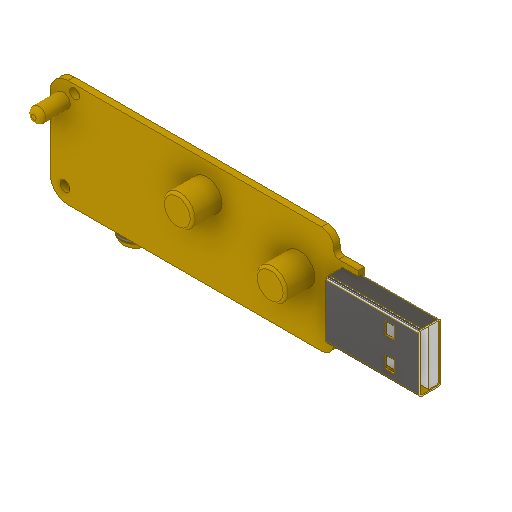
# Autodesk Inventor part: COTS_GENERIC_rtl_sdr_dongle
Saved by Autodesk Inventor 2025 (Build 290162010, 162A)
## iProperties
Created: 2018-09-08
Part Number: COTS_GENERIC_rtl_sdr_dongle
Material: Generic
Document SubType Name: Modeling
Designer: Andrzej
Density: 1 g/cm^3
Appearance: Gold
Author: Andrzej
Autodesk Inventor part; units mm, degrees
ref_plane "YZ Plane" through (0, 0, 0) normal (1, 0, 0) x (0, 1, 0)
ref_plane "XZ Plane" through (0, 0, 0) normal (0, 1, 0) x (-1, 0, 0)
ref_plane "XY Plane" through (0, 0, 0) normal (0, 0, 1) x (1, 0, 0)
sketch "Sketch1" plane through (0, 0, 0) normal (0, 0, 1) x (1, 0, 0)
  line L0 (-11.3863, 5.2126) -> (40.5137, 5.2126)
  line L1 (40.5137, -16.7874) -> (-11.3863, -16.7874)
  line L2 (-14.9863, -13.1874) -> (-14.9863, 1.6126)
  line L3 (44.0137, 1.2126) -> (48.0137, 1.2126)
  line L4 (48.0137, 1.2126) -> (48.0137, -12.7874)
  line L5 (48.0137, -12.7874) -> (44.0137, -12.7874)
  arc A0 (-14.9863, -13.1874) -> (-11.3863, -16.7874) centre (-11.3863, -13.1874) ccw
  arc A1 (-11.3863, 5.2126) -> (-14.9863, 1.6126) centre (-11.3863, 1.6126) ccw
  arc A2 (43.0137, 2.7126) -> (40.5137, 5.2126) centre (40.5137, 2.7126) ccw
  arc A3 (40.5137, -16.7874) -> (43.0137, -14.2874) centre (40.5137, -14.2874) ccw
  line L6 (43.0137, 2.7126) -> (43.0137, 2.2126)
  line L7 (43.0137, -13.7874) -> (43.0137, -14.2874)
  arc A4 (43.0137, 2.2126) -> (44.0137, 1.2126) centre (44.0137, 2.2126) ccw
  arc A5 (44.0137, -12.7874) -> (43.0137, -13.7874) centre (44.0137, -13.7874) ccw
  circle A6 centre (-11.9863, -13.7874) radius 1.05
  circle A7 centre (-9.9863, 3.6126) radius 1.05
  point P0 (0, 0)
  dimension "d3" = 14
  dimension "d4" = 4
  dimension "d7" = 3.6
  dimension "d8" = 2.5
  dimension "d9" = 1
  dimension "d10" = 2.1
  dimension "d11" = 3
  dimension "d12" = 3
  dimension "d13" = 2.1
  dimension "d14" = 5
  dimension "d15" = 1.6
  dimension "d67" = 22
  dimension "d68" = 58
  constraints: 16 end point, 14 tangent, 12 point on circle, 8 centre point, 5 perpendicular, 3 equal radius, 3 parallel, 2 horizontal
  measures "d3" distance of L3.end L4.end
  measures "d4" distance between parallel lines of L0 L3
  measures "d7" radius of A0
  measures "d8" radius of A2
  measures "d9" radius of A4
  measures "d10" diameter of A6
  measures "d11" distance from line of L1 A6.centre
  measures "d12" distance from line of L2 A6.centre
  measures "d13" diameter of A7
  measures "d14" distance from line of L2 A7.centre
  measures "d15" distance from line of L0 A7.centre
  measures "d67" distance between parallel lines of L1 L0
  measures "d68" distance between parallel lines of L2 L6
extrude "Extrusion1" add sketch "Sketch1" along normal blind 1.3
sketch "Sketch2" plane through (0, 0, 1.3) normal (0, 0, 1) x (1, 0, 0)
  circle A0 centre (-9.9863, 3.6126) radius 1.05 projected
  circle A1 centre (-11.9863, -13.7874) radius 1.05 projected
  line L0 (48.0137, 1.2126) -> (44.0137, 1.2126) projected
  arc A2 (43.0137, 2.2126) -> (44.0137, 1.2126) centre (44.0137, 2.2126) ccw projected
  line L1 (43.0137, 2.2126) -> (43.0137, 2.7126) projected
  arc A3 (43.0137, 2.7126) -> (40.5137, 5.2126) centre (40.5137, 2.7126) ccw projected
  line L2 (40.5137, 5.2126) -> (-11.3863, 5.2126) projected
  arc A4 (-11.3863, 5.2126) -> (-14.9863, 1.6126) centre (-11.3863, 1.6126) ccw projected
  line L3 (-14.9863, 1.6126) -> (-14.9863, -13.1874) projected
  arc A5 (-14.9863, -13.1874) -> (-11.3863, -16.7874) centre (-11.3863, -13.1874) ccw projected
  line L4 (-11.3863, -16.7874) -> (40.5137, -16.7874) projected
  arc A6 (40.5137, -16.7874) -> (43.0137, -14.2874) centre (40.5137, -14.2874) ccw projected
  line L5 (43.0137, -14.2874) -> (43.0137, -13.7874) projected
  arc A7 (44.0137, -12.7874) -> (43.0137, -13.7874) centre (44.0137, -13.7874) ccw projected
  line L6 (44.0137, -12.7874) -> (48.0137, -12.7874) projected
  line L7 (48.0137, -12.7874) -> (48.0137, 1.2126) projected
  line L8 (44.8137, 0.2126) -> (44.8137, -11.7874)
  line L9 (44.8137, 0.2126) -> (48.0137, 0.2126)
  line L10 (44.8137, -11.7874) -> (48.0137, -11.7874)
  line L11 (48.0137, -12.7874) -> (48.0137, 1.2126) projected
  line L12 (48.0137, 0.2126) -> (48.0137, -11.7874)
  point P0 (0, 0)
  dimension "d16" = 12
  dimension "d17" = 3.2
  dimension "d18" = 14
  dimension "d19" = 1
  constraints: 8 end point, 2 point on line, 1 collinear, 1 horizontal, 1 perpendicular, 1 vertical
  measures "d16" distance of L8.start L8.end
  measures "d17" distance of L8.start L9.end
  measures "d18" distance between parallel lines of L6 L0
  measures "d19" distance between parallel lines of L0 L9
extrude "Extrusion2" add sketch "Sketch2" along normal blind 3.4 contours L7 L10 L8 L9
sketch "Sketch3" plane through (48.0137, -12.7874, 0) normal (1, 0, 0) x (0, 0, -1)
  line L0 (0, 0) -> (0, 14) projected
  line L1 (0, 14) -> (-1.3, 14) projected
  line L2 (-1.3, 13) -> (-1.3, 14) projected
  line L3 (-1.3, 13) -> (-4.7, 13) projected
  line L4 (-4.7, 1) -> (-4.7, 13) projected
  line L5 (-1.3, 1) -> (-4.7, 1) projected
  line L6 (-1.3, 0) -> (-1.3, 1) projected
  line L7 (0, 0) -> (-1.3, 0) projected
  line L8 (-1.3, 1) -> (-4.7, 1) projected
  line L9 (-1.3, 1) -> (-0.2, 1)
  line L10 (-0.2, 1) -> (-0.2, 13)
  line L11 (-0.2, 13) -> (-1.3, 13)
  point P0 (0, 12.7874)
  dimension "d22" = 4.5
  constraints: 6 end point, 2 perpendicular, 1 horizontal
  measures "d22" distance between parallel lines of L4 L10
extrude "Extrusion3" add sketch "Sketch3" along normal blind 15.8 contours L5 L4 L3 L11 L10 L9
fillet "Fillet1" radius 0.6 4 edges at (54.3137, -11.7874, 4.7) (55.9137, -11.7874, 0.2) (54.3137, 0.2126, 4.7) (55.9137, 0.2126, 0.2)
sketch "Sketch4" plane through (63.8137, -12.7874, 0) normal (1, 0, 0) x (0, 0, -1)
  arc A0 (-0.2, 12.4) -> (-0.8, 13) centre (-0.8, 12.4) ccw projected
  line L0 (-0.8, 13) -> (-4.1, 13) projected
  arc A1 (-4.1, 13) -> (-4.7, 12.4) centre (-4.1, 12.4) ccw projected
  line L1 (-4.7, 12.4) -> (-4.7, 1.6) projected
  arc A2 (-4.7, 1.6) -> (-4.1, 1) centre (-4.1, 1.6) ccw projected
  line L2 (-4.1, 1) -> (-0.8, 1) projected
  arc A3 (-0.8, 1) -> (-0.2, 1.6) centre (-0.8, 1.6) ccw projected
  line L3 (-0.2, 1.6) -> (-0.2, 12.4) projected
  line L4 (-4.4, 1.6) -> (-4.4, 12.4)
  arc A4 (-4.1, 12.7) -> (-4.4, 12.4) centre (-4.1, 12.4) ccw
  line L5 (-4.1, 12.7) -> (-0.8, 12.7)
  arc A5 (-0.5, 12.4) -> (-0.8, 12.7) centre (-0.8, 12.4) ccw
  line L6 (-0.5, 12.4) -> (-0.5, 1.6)
  arc A6 (-0.8, 1.3) -> (-0.5, 1.6) centre (-0.8, 1.6) ccw
  line L7 (-0.8, 1.3) -> (-4.1, 1.3)
  arc A7 (-4.4, 1.6) -> (-4.1, 1.3) centre (-4.1, 1.6) ccw
  line L8 (-2.45, 1.3) -> (-2.45, 12.7)
  point P0 (0, 12.7874)
  dimension "d26" = 0.3
  constraints: 10 end point, 8 point on circle, 4 centre point, 2 midpoint, 7 other
  measures "d26" distance between parallel lines of L1 L4
extrude "Extrusion4" cut sketch "Sketch4" against normal blind 15 contours L4 A4 L5 L8 L7 A7
sketch "Sketch5" plane through (0, 0, 0) normal (0, 0, -1) x (-1, 0, 0)
  line L0 (2.5863, -9.5874) -> (8.5863, -9.5874)
  line L1 (8.5863, -9.5874) -> (8.5863, -15.5874)
  line L2 (8.5863, -15.5874) -> (2.5863, -15.5874)
  line L3 (2.5863, -15.5874) -> (2.5863, -9.5874)
  line L4 (14.9863, 1.6126) -> (14.9863, -13.1874) projected
  line L5 (-40.5137, 5.2126) -> (11.3863, 5.2126) projected
  point P0 (0, 0)
  dimension "d29" = 6
  dimension "d30" = 6
  dimension "d31" = 6.4
  dimension "d32" = 14.8
  constraints: 8 end point, 2 parallel, 1 horizontal, 1 perpendicular
  measures "d29" distance of L1.end L2.end
  measures "d30" distance of L0.end L1.end
  measures "d31" distance between parallel lines of L4 L1
  measures "d32" distance between parallel lines of L5 L0
extrude "Extrusion5" add sketch "Sketch5" along normal blind 10
sketch "Sketch6" plane through (-8.5863, -15.5874, 0) normal (0, -1, 0) x (1, 0, 0)
  line L0 (0, 0) -> (6, 0) projected
  line L1 (0, 0) -> (0, -10) projected
  line L2 (6, -10) -> (0, -10) projected
  line L3 (6, 0) -> (6, -10) projected
  circle A0 centre (3, -6.95) radius 2.65
  point P0 (8.5863, 0)
  dimension "d35" = 5.3
  dimension "d36" = 3.05
  dimension "d37" = 6.95
  constraints: 1 centre point
  measures "d35" diameter of A0
  measures "d36" distance from line of L2 A0.centre
  measures "d37" distance from line of L0 A0.centre
extrude "Extrusion6" add sketch "Sketch6" along normal blind 3.3 contours A0
sketch "Sketch7" plane through (-5.5863, -18.8874, -6.95) normal (0, -1, 0) x (1, 0, 0)
  circle A0 centre (0, 0) radius 3.15
  point P0 (5.5863, 6.95)
  dimension "d40" = 6.3
  constraints: 1 centre point
  measures "d40" diameter of A0
extrude "Extrusion7" add sketch "Sketch7" along normal blind 4
sketch "Sketch8" plane through (-5.5863, -22.8874, -6.95) normal (0, -1, 0) x (1, 0, 0)
  circle A0 centre (0, 0) radius 2.65 projected
  point P0 (5.5863, 6.95)
extrude "Extrusion8" add sketch "Sketch8" along normal blind 1
thread "Thread1" size "M7x0.5" class "6g" standard "ANSI Metric M Profile" full length
sketch "Sketch9" plane through (-5.5863, -23.8874, -6.95) normal (0, -1, 0) x (1, 0, 0)
  circle A0 centre (0, 0) radius 2.65 projected
  circle A1 centre (0, 0) radius 2.35
  point P0 (5.5863, 6.95)
  dimension "d47" = 0.3
  constraints: 1 centre point
  measures "d47" radial gap between concentric circles of A0 A1
extrude "Extrusion9" cut sketch "Sketch9" against normal blind 2 contours A1
fillet "Fillet2" radius 0.25 4 edges at (-2.5863, -15.5874, -5) (-2.5863, -9.5874, -5) (-8.5863, -15.5874, -5) (-8.5863, -9.5874, -5)
fillet "Fillet2" radius 0.5 4 edges at (-2.5863, -12.5874, -10) (-5.5863, -15.5874, -10) (-8.5863, -12.5874, -10) (-5.5863, -9.5874, -10)
sketch "Sketch10" plane through (0, 0, 1.3) normal (0, 0, 1) x (1, 0, 0)
  circle A0 centre (17.0137, -0.7874) radius 3.15
  circle A1 centre (36.0137, -4.3874) radius 3.15
  line L0 (48.0137, -11.7874) -> (44.8137, -11.7874) projected
  line L1 (44.8137, -11.7874) -> (44.8137, 0.2126) projected
  line L2 (44.8137, 0.2126) -> (48.0137, 0.2126) projected
  line L3 (48.0137, 0.2126) -> (48.0137, 1.2126) projected
  line L4 (48.0137, 1.2126) -> (44.0137, 1.2126) projected
  arc A2 (43.0137, 2.2126) -> (44.0137, 1.2126) centre (44.0137, 2.2126) ccw projected
  line L5 (43.0137, 2.2126) -> (43.0137, 2.7126) projected
  arc A3 (43.0137, 2.7126) -> (40.5137, 5.2126) centre (40.5137, 2.7126) ccw projected
  line L6 (40.5137, 5.2126) -> (-11.3863, 5.2126) projected
  arc A4 (-11.3863, 5.2126) -> (-14.9863, 1.6126) centre (-11.3863, 1.6126) ccw projected
  line L7 (-14.9863, 1.6126) -> (-14.9863, -13.1874) projected
  arc A5 (-14.9863, -13.1874) -> (-11.3863, -16.7874) centre (-11.3863, -13.1874) ccw projected
  line L8 (-11.3863, -16.7874) -> (40.5137, -16.7874) projected
  arc A6 (40.5137, -16.7874) -> (43.0137, -14.2874) centre (40.5137, -14.2874) ccw projected
  line L9 (43.0137, -14.2874) -> (43.0137, -13.7874) projected
  arc A7 (44.0137, -12.7874) -> (43.0137, -13.7874) centre (44.0137, -13.7874) ccw projected
  line L10 (44.0137, -12.7874) -> (48.0137, -12.7874) projected
  line L11 (48.0137, -12.7874) -> (48.0137, -11.7874) projected
  circle A8 centre (-11.9863, -13.7874) radius 1.05 projected
  circle A9 centre (-9.9863, 3.6126) radius 1.05 projected
  circle A10 centre (-12.3863, 1.2126) radius 1.5
  point P0 (0, 0)
  dimension "d52" = 6.3
  dimension "d53" = 6.3
  dimension "d54" = 7
  dimension "d55" = 9.6
  dimension "d56" = 32
  dimension "d57" = 6
  dimension "d61" = 3
  dimension "d62" = 2.6
  dimension "d63" = 4
  constraints: 3 centre point
  measures "d52" diameter of A0
  measures "d53" diameter of A1
  measures "d54" horizontal distance of L5.end A1.centre
  measures "d55" distance from line of L6 A1.centre
  measures "d56" distance from line of L7 A0.centre
  measures "d57" distance from line of L6 A0.centre
  measures "d61" diameter of A10
  measures "d62" distance from line of L7 A10.centre
  measures "d63" distance from line of L6 A10.centre
extrude "Extrusion10" add sketch "Sketch10" along normal blind 6 contours A0 | A1
fillet "Fillet3" radius 0.5 2 edges at (13.8637, -0.7874, 7.3) (32.8637, -4.3874, 7.3)
extrude "Extrusion11" add sketch "Sketch10" along normal blind 6 contours A10
fillet "Fillet4" radius 1 1 edges at (-13.8863, 1.2126, 7.3)
sketch "Sketch11" plane through (0, 0, 4.7) normal (0, 0, 1) x (1, 0, 0)
  line L0 (56.9137, -10.0086) -> (58.8137, -10.0086)
  line L1 (58.8137, -10.0086) -> (58.8137, -7.5086)
  line L2 (58.8137, -7.5086) -> (56.9137, -7.5086)
  line L3 (56.9137, -7.5086) -> (56.9137, -10.0086)
  line L4 (63.8137, -0.3874) -> (63.8137, -11.1874) projected
  line L5 (56.9137, -4.0086) -> (58.8137, -4.0086)
  line L6 (58.8137, -4.0086) -> (58.8137, -1.5086)
  line L7 (58.8137, -1.5086) -> (56.9137, -1.5086)
  line L8 (56.9137, -1.5086) -> (56.9137, -4.0086)
  point P0 (0, 0)
  dimension "d69" = 1.9
  dimension "d70" = 2.5
  dimension "d71" = 5
  dimension "d72" = 1.9
  dimension "d73" = 2.5
  dimension "d74" = 5
  dimension "d75" = 3.5
  constraints: 16 end point, 4 parallel, 2 horizontal, 2 perpendicular
  measures "d69" distance of L2.end L1.end
  measures "d70" distance of L1.end L0.end
  measures "d71" distance between parallel lines of L4 L1
  measures "d72" distance of L7.end L6.end
  measures "d73" distance of L6.end L5.end
  measures "d74" distance between parallel lines of L6 L4
  measures "d75" distance between parallel lines of L5 L2
extrude "Extrusion12" cut sketch "Sketch11" against normal blind 1
extrude "Extrusion13" cut sketch "Sketch4" against normal blind 0.2 contours L8 L5 A5 L6 A6 L7
equation "\"d4\" = -0.5 * d3 + 0.5 * d1"
equation "\"d19\" = -0.5 * d16 + 0.5 * d18"
equation "\"d74\" = d71"
equation "\"d1\" = 22"
body "Solid1"
